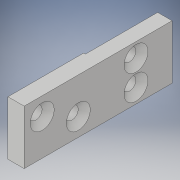
# Autodesk Inventor part: SidePlateRight
Saved by Autodesk Inventor 2019 (Build 230136000, 136)
## iProperties
Created: 2019-09-28
Part Number: SidePlateRight
Material: Generic
Document SubType Name: Modeling
Designer: james
Density: 1 g/cm^3
Appearance: Default
Author: james
Autodesk Inventor part; units mm, degrees
ref_plane "YZ Plane" through (0, 0, 0) normal (1, 0, 0) x (0, 1, 0)
ref_plane "XZ Plane" through (0, 0, 0) normal (0, 1, 0) x (-1, 0, 0)
ref_plane "XY Plane" through (0, 0, 0) normal (0, 0, 1) x (1, 0, 0)
sketch "Sketch1" plane through (0, 0, 0) normal (1, 0, 0) x (0, 1, 0)
  line L0 (7.5884, 18.4529) -> (-11.4616, 18.4529)
  line L1 (-11.4616, 18.4529) -> (-11.4616, -33.6171)
  line L2 (-11.4616, -33.6171) -> (7.5884, -33.6171)
  line L3 (7.5884, -33.6171) -> (7.5884, 18.4529)
  point P0 (0, 0)
  dimension "d0" = 52.07
  dimension "d1" = 19.05
  constraints: 8 end point, 2 parallel, 1 horizontal, 1 perpendicular
  measures "d0" distance of L2.end L0.start
  measures "d1" distance of L0.start L0.end
extrude "Extrusion1" add sketch "Sketch1" along normal blind 6.35
sketch "Sketch3" plane through (0, 7.5884, 18.4529) normal (0, 1, 0) x (1, 0, 0)
  line L0 (0, 26.67) -> (0.635, 26.67)
  line L1 (0.635, 26.67) -> (0.635, 52.07)
  line L2 (0.635, 52.07) -> (0, 52.07)
  line L3 (0, 52.07) -> (0, 26.67)
  line L4 (5.715, 52.07) -> (6.35, 52.07)
  line L5 (6.35, 52.07) -> (6.35, 26.67)
  line L6 (6.35, 26.67) -> (5.715, 26.67)
  line L7 (5.715, 26.67) -> (5.715, 52.07)
  line L8 (6.35, 52.07) -> (6.35, 0) projected
  line L9 (0, 52.07) -> (0, 0) projected
  line L10 (0, 52.07) -> (6.35, 52.07) projected
  point P0 (0, 18.4529)
  dimension "d19" = 25.4
  dimension "d20" = 25.4
  dimension "d21" = 0
  dimension "d22" = 0
  dimension "d23" = 0.635
  dimension "d24" = 0.635
  dimension "d25" = 0
  constraints: 16 end point, 4 parallel, 2 horizontal, 2 perpendicular, 1 point on line
  measures "d19" distance of L0.end L1.end
  measures "d20" distance of L6.end L4.start
  measures "d21" distance between parallel lines of L8 L5
  measures "d22" distance between parallel lines of L9 L3
  measures "d23" distance of L0.start L0.end
  measures "d24" distance of L5.end L6.end
  measures "d25" distance between parallel lines of L10 L4
extrude "Extrusion2" cut sketch "Sketch3" against normal blind 50.8
sketch "Sketch6" plane through (5.715, 7.5884, -8.2171) normal (1, 0, 0) x (0, 0, -1)
  line L0 (0, 0) -> (25.4, 0) projected
  line L1 (25.4, 0) -> (25.4, -19.05) projected
  point P0 (-8.2171, -7.5884)
  point P1 (12.7, -5.08)
  point P2 (12.7, -13.97)
  dimension "d39" = 5.08
  dimension "d40" = 13.97
  dimension "d41" = 12.7
  dimension "d42" = 12.7
  measures "d39" distance from line of L0 point (12.7, -5.08)
  measures "d40" distance from line of L0 point (12.7, -13.97)
  measures "d41" distance from line of L1 point (12.7, -5.08)
  measures "d42" distance from line of L1 point (12.7, -13.97)
hole "Hole3" at (5.715, 2.5084, -20.9171) at (5.715, -6.3816, -20.9171) direction (-1, 0, 0) diameter 4.4958 end through all countersink diameter 8.4328 countersink angle 82 clearance for "Flat Head Machine Screw (82)" size "#8" standard "Ansi Unified Screw Threads"
sketch "Sketch7" plane through (0, 7.5884, 18.4529) normal (0, 1, 0) x (1, 0, 0)
  line L0 (8.7509, 0) -> (5.715, 0)
  line L1 (5.715, 0) -> (5.715, 29.619)
  line L2 (5.715, 29.619) -> (8.7509, 29.619)
  line L3 (8.7509, 29.619) -> (8.7509, 0)
  line L4 (5.715, 26.67) -> (5.715, 52.07) projected
  line L5 (0, 0) -> (6.35, 0) projected
  point P0 (0, 18.4529)
  dimension "d50" = 0
  dimension "d51" = 0
  constraints: 8 end point, 2 parallel, 1 horizontal, 1 perpendicular
  measures "d50" distance between parallel lines of L4 L1
  measures "d51" distance between parallel lines of L5 L0
extrude "Extrusion3" cut sketch "Sketch7" against normal blind 25.4
sketch "Sketch8" plane through (5.715, 7.5884, 18.4529) normal (1, 0, 0) x (0, 0, -1)
  line L0 (0, 0) -> (52.07, 0) projected
  line L1 (0, -19.05) -> (0, 0) projected
  point P0 (18.4529, -7.5884)
  point P1 (6.35, -6.35)
  point P2 (19.05, -12.7)
  dimension "d54" = 6.35
  dimension "d55" = 6.35
  dimension "d56" = 19.05
  dimension "d57" = 12.7
  measures "d54" distance from line of L0 point (6.35, -6.35)
  measures "d55" distance from line of L1 point (6.35, -6.35)
  measures "d56" distance from line of L1 point (19.05, -12.7)
  measures "d57" distance from line of L0 point (19.05, -12.7)
hole "Hole4" at (5.715, 1.2384, 12.1029) at (5.715, -5.1116, -0.5971) direction (-1, 0, 0) diameter 4.4958 end through all countersink diameter 8.4328 countersink angle 82 clearance for "Flat Head Machine Screw (82)" size "#8" standard "Ansi Unified Screw Threads"
body "Solid1"
